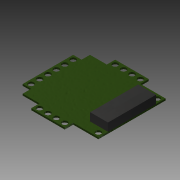
# Autodesk Inventor part: legoduino
Saved by Autodesk Inventor 2013 (Build 170138000, 138)
## iProperties
Created: 2013-10-21
Part Number: legoduino
Material: Generic
Document SubType Name: Modeling
Designer: Masta
Density: 1 g/cm^3
Author: Masta
Autodesk Inventor part; units mm, degrees
ref_plane "YZ Plane" through (0, 0, 0) normal (1, 0, 0) x (0, 1, 0)
ref_plane "XZ Plane" through (0, 0, 0) normal (0, 1, 0) x (-1, 0, 0)
ref_plane "XY Plane" through (0, 0, 0) normal (0, 0, 1) x (1, 0, 0)
sketch "Sketch1" plane through (0, 0, 0) normal (0, 0, 1) x (1, 0, 0)
  line L0 (0, 0) -> (-40, 0)
  line L1 (-40, 0) -> (-40, 24)
  line L2 (-40, 24) -> (-32, 24)
  line L3 (-32, 24) -> (-32, 32)
  line L4 (-32, 32) -> (-16, 32)
  line L5 (-16, 32) -> (-16, 40)
  line L6 (-16, 40) -> (16, 40)
  line L7 (16, 40) -> (16, 32)
  line L8 (16, 32) -> (40, 32)
  line L9 (40, 32) -> (40, 0)
  line L10 (40, 0) -> (0, 0)
  line L11 (-36, 0) -> (-36, 24) construction
  line L12 (-16, 36) -> (16, 36) construction
  circle A0 centre (-36, 20) radius 2.6
  circle A1 centre (-36, 12) radius 2.6
  circle A2 centre (-36, 4) radius 2.6
  circle A3 centre (36, 28) radius 2.6
  circle A4 centre (-12, 36) radius 2.6
  circle A5 centre (-4, 36) radius 2.6
  circle A6 centre (4, 36) radius 2.6
  circle A7 centre (12, 36) radius 2.6
  line L13 (40, 22.86) -> (23, 22.86)
  line L14 (23, 22.86) -> (23, 0)
  dimension "d0" = 40
  dimension "d1" = 24
  dimension "d2" = 8
  dimension "d3" = 8
  dimension "d4" = 16
  dimension "d5" = 8
  dimension "d6" = 32
  dimension "d7" = 8
  dimension "d8" = 24
  dimension "d9" = 5.2
  dimension "d10" = 4
  dimension "d11" = 8
  dimension "d12" = 4
  dimension "d13" = 4
  dimension "d14" = 4
  dimension "d15" = 4
  dimension "d16" = 8
  dimension "d17" = 8
  dimension "d18" = 8
  dimension "d21" = 17
  dimension "d22" = 22.86
  constraints: 30 end point, 10 point on line, 8 centre point, 7 equal radius, 6 perpendicular, 5 parallel, 4 midpoint, 1 collinear, 1 horizontal, 1 vertical
  measures "d0" distance of L0.start L0.end
  measures "d1" distance of L0.end L1.end
  measures "d2" distance of L1.end L2.end
  measures "d3" distance of L2.end L3.end
  measures "d4" distance of L3.end L4.end
  measures "d5" distance of L4.end L5.end
  measures "d6" distance of L5.end L6.end
  measures "d7" distance of L6.end L7.end
  measures "d8" distance of L7.end L8.end
  measures "d9" diameter of A0
  measures "d10" distance from line of L2 A0.centre
  measures "d11" distance of A0.centre A1.centre
  measures "d12" distance from line of L0 A2.centre
  measures "d13" distance from line of L8 A3.centre
  measures "d14" distance from line of L9 A3.centre
  measures "d15" distance from line of L7 A7.centre
  measures "d16" distance of A6.centre A7.centre
  measures "d17" distance of A5.centre A6.centre
  measures "d18" distance of A4.centre A5.centre
  measures "d21" distance of L13.start L13.end
  measures "d22" distance of L13.end L14.end
extrude "Extrusion1" add sketch "Sketch1" against normal blind 1.6
extrude "Extrusion2" add sketch "Sketch1" along normal blind 7.62 separate body contours L14 L13 L9 L10
mirror "Mirror1" about plane through (0, 0, 0) normal (0, -1, 0) of "Extrusion1" bodies 1
mirror "Mirror2" about plane through (23, 0, 0) normal (0, -1, 0) of "Extrusion2" bodies 2
body "Solid1"
body "Solid2"
